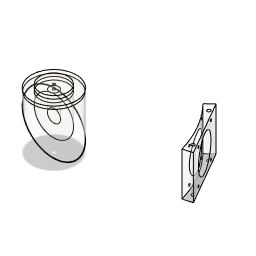
cage v11 (Autodesk Fusion 360 design; units mm, degrees)
Autodesk Fusion 360 part; units mm, degrees
note: some values were not read from the file. Chosen so that the rebuilt part matches the saved one: which bodies a step acts on; which face or edge a step refers to. Set by a fixed rule: which sketch regions a step uses.
(part 1 of 2)
sketch "Plate" plane through (0, 0, 0) normal (0, 1, 0) x (1, 0, 0) in component "Top Plate"
  circle A0 centre (0, 0) radius 228.6
  line L0 (0, 260.35) -> (0, 228.6) construction
  arc A1 (-273.05, -164.9615) -> (273.05, -164.9615) centre (0, 125.8796) ccw
  line L1 (-273.05, -164.9615) -> (-273.05, 0)
  line L2 (273.05, -164.9615) -> (273.05, 0)
  line L3 (0, 307.975) -> (126.2968, 242.0856)
  line L4 (0, 307.975) -> (-126.2968, 242.0856)
  circle A2 centre (0, 260.35) radius 3.302
  circle A3 centre (0, 0) radius 260.35 construction
  circle A4 centre (0, 260.35) radius 22.225 construction
  line L5 (0, -228.6) -> (0, -273.05) construction
  circle A5 centre (0, 0) radius 269.875 construction
  circle A6 centre (234.95, -132.7818) radius 22.225 construction
  circle A7 centre (234.95, -132.7818) radius 3.302
  circle A8 centre (-234.95, -132.7818) radius 3.302
  circle A9 centre (-234.95, -132.7818) radius 22.225 construction
  line L6 (-234.95, -132.7818) -> (234.95, -132.7818) construction
  arc A10 (-126.2968, 242.0856) -> (-273.05, 0) centre (0, 0) ccw
  arc A11 (273.05, 0) -> (126.2968, 242.0856) centre (0, 0) ccw
  line L7 (0, -228.6) -> (0, 0) construction
  line L8 (0, 0) -> (0, 228.6) construction
  line L9 (0, 260.35) -> (0, 307.975) construction
  line L10 (-126.2968, 242.0856) -> (126.2968, 242.0856) construction
  line L11 (-273.05, -164.9615) -> (0, 307.975) construction
  circle A12 centre (0, 0) radius 250.825 construction
  circle A13 centre (191.5577, 161.9223) radius 3.302
  circle A14 centre (236.0077, 84.9327) radius 3.302
  line L12 (191.5577, 161.9223) -> (236.0077, 84.9327) construction
  circle A15 centre (-236.0077, 84.9327) radius 3.302
  line L13 (-191.5577, 161.9223) -> (-236.0077, 84.9327) construction
  circle A16 centre (-191.5577, 161.9223) radius 3.302
  circle A17 centre (44.45, -246.855) radius 3.302
  line L14 (-44.45, -246.855) -> (44.45, -246.855) construction
  circle A18 centre (-44.45, -246.855) radius 3.302
  line L15 (213.7827, 123.4275) -> (0, -246.855) construction
  line L16 (0, -246.855) -> (-213.7827, 123.4275) construction
  line L17 (-213.7827, 123.4275) -> (213.7827, 123.4275) construction
  point P0 (0, -246.855)
  point P1 (-213.7827, 123.4275)
  point P2 (213.7827, 123.4275)
  dimension "d16_2" = 457.2
  dimension "d19_2" = 546.1
  dimension "d22_2" = 79.375
  dimension "d24_2" = 31.75
  dimension "d160_1" = 539.75
  dimension "d162_1" = 6.604
  dimension "d163_1" = 6.604
  dimension "d164_1" = 469.9
  dimension "d165_1" = 44.45
  dimension "d166_1" = 44.45
  dimension "d167_1" = 44.45
  dimension "d168_1" = 44.45
  dimension "d169_1" = 546.1
  dimension "d171_1" = 501.65
  dimension "d172_1" = 6.604
  dimension "d174_1" = 6.604
  dimension "d175_1" = 88.9
  dimension "d176_1" = 6.604
  dimension "d177_1" = 6.604
  dimension "d178_1" = 88.9
  dimension "d179_1" = 6.604
  dimension "d180_1" = 6.604
  dimension "d181_1" = 88.9
  dimension "d350" = 6.604
  constraint coincident A0.centre A3.centre
  constraint coincident A0 L0.end
  constraint vertical L0
  constraint concentric A0 A3
  constraint coincident L0.start A3
  constraint coincident A0 L5.start
  constraint midpoint A1 L5.end
  constraint vertical L5
  constraint coincident A5 A6.centre
  constraint concentric A6 A7
  constraint concentric A8 A9
  constraint coincident A8.centre A9.centre
  constraint coincident A6.centre A7.centre
  constraint horizontal L6
  constraint coincident A5 A8.centre
  constraint vertical L1
  constraint vertical L2
  constraint tangent L4 A10
  constraint tangent L3 A11
  constraint vertical L7
  constraint coincident L0.start A2.centre
  constraint vertical L9
  constraint collinear L0 L8
  constraint horizontal L10
  constraint tangent L1 A10
  constraint concentric A5 A12
  constraint coincident A12 A13.centre
  constraint coincident A12 A14.centre
  constraint coincident A13.centre L12.start
  constraint coincident A14.centre L12.end
  constraint coincident L13.start A16.centre
  constraint coincident A15.centre L13.end
  constraint coincident L14.start A18.centre
  constraint coincident A17.centre L14.end
  constraint coincident A12 A15.centre
  constraint coincident A12 L13.start
  constraint coincident A12 A17.centre
  constraint coincident A12 L14.start
  constraint midpoint L14 P0
  constraint coincident L5 P0
  constraint midpoint L13 P1
  constraint midpoint L12 P2
  constraint coincident P2 L15.start
  constraint coincident P0 L15.end
  constraint coincident P1 L16.end
  constraint equal L16 L17
  constraint equal L15 L16
  measures "d16_2" diameter of A0
  measures "d19_2" distance of A1.start A1.end
  measures "d22_2" distance of L3.start L0.end
  measures "d24_2" distance of L0.end L0.start
  measures "d160_1" diameter of A5
  measures "d162_1" diameter of A7
  measures "d163_1" diameter of A8
  measures "d164_1" distance of A8.centre A6.centre
  measures "d165_1" diameter of A9
  measures "d166_1" diameter of A6
  measures "d167_1" distance of L5.start L5.end
  measures "d168_1" diameter of A4
  measures "d169_1" distance of A1.start L3.start
  measures "d171_1" diameter of A12
  measures "d172_1" diameter of A13
  measures "d174_1" diameter of A14
  measures "d175_1" distance of A13.centre A14.centre
  measures "d176_1" diameter of A16
  measures "d177_1" diameter of A15
  measures "d178_1" distance of L13.start A15.centre
  measures "d179_1" diameter of A18
  measures "d180_1" diameter of A17
  measures "d181_1" distance of L14.start A17.centre
  measures "d350" diameter of A2
extrude "Extrude4" add sketch "Plate" along normal blind 19.05 makes body 1 in component "Top Plate"
sketch "Sketch1" plane through (0, 0, 0) normal (1, 0, 0) x (0, 0, -1) in component "Slice1"
  line L0 (-339.5498, 170.2069) -> (354.2377, 170.2069)
  line L1 (354.2377, 170.2069) -> (354.2377, -114.9113)
  line L2 (354.2377, -114.9113) -> (-339.5498, -114.9113)
  line L3 (-339.5498, -114.9113) -> (-339.5498, 170.2069)
  constraint horizontal L0
  constraint vertical L1
  constraint horizontal L2
  constraint vertical L3
extrude "Extrude1" add sketch "Sketch1" along normal blind 228.6 separate body makes body 2 in component "Slice1"
sketch "Sketch1 (2)" plane through (0, 0, 0) normal (1, 0, 0) x (0, 0, -1) in component "Slice2"
  line L0 (-339.5498, 170.2069) -> (354.2377, 170.2069)
  line L1 (354.2377, 170.2069) -> (354.2377, -114.9113)
  line L2 (354.2377, -114.9113) -> (-339.5498, -114.9113)
  line L3 (-339.5498, -114.9113) -> (-339.5498, 170.2069)
  constraint horizontal L0
  constraint vertical L1
  constraint horizontal L2
  constraint vertical L3
extrude "Extrude1'" add sketch "Sketch1 (2)" along normal blind 177.8 separate body makes body 3 in component "Slice2"
split "Split3" by plane through (0, 0, 0) normal (0.707107, 0, 0.707107) bodies 1 makes body 4 at (56.2654, 0, -258.2251) in component "Top Plate"
split "Split4" by plane through (0, 0, 0) normal (0.707107, 0, -0.707107) bodies 4 1 makes body 6 at (178.8171, 0, 204.0038) makes body 5 at (-261.2405, 0, 98.6008) in component "Top Plate"
copy_body "Body->Comp5" bodies 1 removing the originals makes body 7 in component "right (1)"
copy_body "Body->Comp6" bodies 4 removing the originals makes body 8 in component "front (1)"
copy_body "Body->Comp7" bodies 6 removing the originals makes body 9 in component "rear (1)"
copy_body "Body->Comp8" bodies 5 removing the originals makes body 10 in component "left (1)"
split "Split1" by plane through (0, 0, 0) normal (1, 0, 0) bodies 9 makes body 11 at (171.3232, 0, 210.5758) in component "rear (1)"
copy_body "Body->Comp1" bodies 9 removing the originals makes body 12 in component "left (2)"
copy_body "Body->Comp2" bodies 11 removing the originals makes body 13 in component "right (2)"
sketch "Sketch1 (3)" plane through (0, 0, 0) normal (1, 0, 0) x (0, 0, -1) in component "left (2)"
  line L0 (-273.05, 0) -> (-228.6, 0)
  line L1 (-228.6, 0) -> (-228.6, 19.05)
  line L2 (-228.6, 19.05) -> (-273.05, 19.05)
  line L3 (-273.05, 19.05) -> (-273.05, 0)
  line L4 (-266.7, 12.7) -> (-234.95, 12.7)
  line L5 (-234.95, 12.7) -> (-234.95, 6.35)
  line L6 (-234.95, 6.35) -> (-266.7, 6.35)
  line L7 (-266.7, 6.35) -> (-266.7, 12.7)
  line L8 (-256.54, 12.7) -> (-256.54, 19.05) construction
  line L9 (-241.3, 6.35) -> (-241.3, 0) construction
  line L10 (-234.95, 10.16) -> (-228.6, 10.16) construction
  line L11 (-266.7, 7.62) -> (-273.05, 7.62) construction
  dimension "d194" = 6.35
  dimension "d195" = 6.35
  dimension "d196" = 31.75
  dimension "d197" = 6.35
  constraint horizontal L4
  constraint vertical L5
  constraint horizontal L6
  constraint vertical L7
  constraint coincident L4 L8.start
  constraint coincident L2 L8.end
  constraint perpendicular L2 L8
  constraint coincident L6 L9.start
  constraint coincident L0 L9.end
  constraint perpendicular L0 L9
  constraint coincident L5 L10.start
  constraint coincident L1 L10.end
  constraint perpendicular L1 L10
  constraint coincident L7 L11.start
  constraint coincident L3 L11.end
  constraint perpendicular L3 L11
  constraint equal L10 L11
  constraint equal L8 L9
  measures "d194" distance of L8.start L8.end
  measures "d195" distance of L10.start L10.end
  measures "d196" distance of L5.end L6.end
  measures "d197" distance of L4.end L5.end
extrude "Extrude1''" cut sketch "Sketch1 (3)" against normal blind 12.7 contours L4 L5 L6 L7 bodies 12 in component "left (2)"
sketch "Sketch1 (4)" plane through (0, 0, 0) normal (-1, 0, 0) x (0, 0, 1) in component "right (2)"
  line L0 (228.6, 0) -> (273.05, 0)
  line L1 (273.05, 0) -> (273.05, 19.05)
  line L2 (273.05, 19.05) -> (228.6, 19.05)
  line L3 (228.6, 19.05) -> (228.6, 0)
  line L4 (234.95, 12.7) -> (266.7, 12.7)
  line L5 (266.7, 12.7) -> (266.7, 6.35)
  line L6 (266.7, 6.35) -> (234.95, 6.35)
  line L7 (234.95, 6.35) -> (234.95, 12.7)
  line L8 (240.9533, 6.35) -> (240.9533, 0) construction
  line L9 (256.54, 12.7) -> (256.54, 19.05) construction
  line L10 (266.7, 6.1597) -> (273.05, 6.1597) construction
  line L11 (234.95, 11.1721) -> (228.6, 11.1721) construction
  dimension "d200" = 6.35
  dimension "d201" = 6.35
  dimension "d202" = 31.75
  dimension "d203" = 6.35
  constraint horizontal L4
  constraint vertical L5
  constraint horizontal L6
  constraint vertical L7
  constraint coincident L6 L8.start
  constraint coincident L0 L8.end
  constraint perpendicular L0 L8
  constraint coincident L4 L9.start
  constraint coincident L2 L9.end
  constraint perpendicular L2 L9
  constraint coincident L5 L10.start
  constraint coincident L1 L10.end
  constraint perpendicular L1 L10
  constraint coincident L7 L11.start
  constraint coincident L3 L11.end
  constraint perpendicular L3 L11
  constraint equal L10 L11
  constraint equal L8 L9
  measures "d200" distance of L11.start L11.end
  measures "d201" distance of L8.start L8.end
  measures "d202" distance of L4.start L4.end
  measures "d203" distance of L4.start L6.end
extrude "Extrude1'''" cut sketch "Sketch1 (4)" against normal blind 12.7 contours L4 L5 L6 L7 bodies 13 in component "right (2)"
sketch "Sketch1 (5)" plane through (0, 6.35, 0) normal (0, 1, 0) x (-1, 0, 0) in component "Connector"
  line L0 (0, 266.7) -> (0, 234.95)
  line L1 (0, 234.95) -> (12.7, 234.95)
  line L2 (12.7, 234.95) -> (12.7, 266.7)
  line L3 (12.7, 266.7) -> (0, 266.7)
  line L4 (12.7, 266.192) -> (-12.192, 266.192)
  line L5 (-12.192, 266.192) -> (-12.192, 234.95)
  line L6 (-12.192, 234.95) -> (12.7, 234.95)
  line L7 (12.7, 234.95) -> (12.7, 266.192)
  dimension "d206" = 31.242
  dimension "d207" = 24.892
  constraint horizontal L4
  constraint vertical L5
  constraint horizontal L6
  constraint vertical L7
  constraint coincident L1.end L2.start
  measures "d206" distance of L1.end L4.start
  measures "d207" distance of L1.end L5.end
extrude "Extrude1''''" add sketch "Sketch1 (5)" along normal blind 5.715 separate body contours L0 L1 L2 L4 L6 L7 | L0 L4 L5 L6 makes body 14 in component "Connector"
sketch "Sketch2" plane through (0, 0, 0) normal (0.707107, 0, -0.707107) x (-0.707107, 0, -0.707107) in component "right (2)"
  line L0 (-228.6, 19.05) -> (-299.8624, 19.05)
  line L1 (-299.8624, 19.05) -> (-299.8624, 0)
  line L2 (-299.8624, 0) -> (-228.6, 0)
  line L3 (-228.6, 0) -> (-228.6, 19.05)
  line L4 (-293.5124, 12.7) -> (-234.95, 12.7)
  line L5 (-234.95, 12.7) -> (-234.95, 6.35)
  line L6 (-234.95, 6.35) -> (-293.5124, 6.35)
  line L7 (-293.5124, 6.35) -> (-293.5124, 12.7)
  line L8 (-276.86, 12.7) -> (-276.86, 19.05) construction
  line L9 (-293.5124, 9.3745) -> (-299.8624, 9.3745) construction
  line L10 (-248.92, 6.35) -> (-248.92, 0) construction
  line L11 (-234.95, 7.62) -> (-228.6, 7.62) construction
  dimension "d210" = 6.35
  dimension "d211" = 6.35
  constraint horizontal L4
  constraint vertical L5
  constraint horizontal L6
  constraint vertical L7
  constraint coincident L4 L8.start
  constraint coincident L0 L8.end
  constraint perpendicular L4 L8
  constraint coincident L7 L9.start
  constraint coincident L1 L9.end
  constraint perpendicular L1 L9
  constraint coincident L6 L10.start
  constraint coincident L2 L10.end
  constraint perpendicular L2 L10
  constraint coincident L5 L11.start
  constraint coincident L3 L11.end
  constraint perpendicular L3 L11
  constraint equal L9 L11
  constraint equal L8 L10
  measures "d210" distance of L8.start L8.end
  measures "d211" distance of L9.start L9.end
extrude "Extrude2" cut sketch "Sketch2" against normal blind 12.7 contours L4 L5 L6 L7 bodies 13 in component "right (2)"
sketch "Sketch3" plane through (0, 0, 0) normal (-0.707107, 0, -0.707107) x (-0.707107, 0, 0.707107) in component "left (2)"
  line L0 (299.8624, 0) -> (299.8624, 19.05)
  line L1 (299.8624, 19.05) -> (228.6, 19.05)
  line L2 (228.6, 19.05) -> (228.6, 0)
  line L3 (228.6, 0) -> (299.8624, 0)
  line L4 (234.95, 12.7) -> (293.5124, 12.7)
  line L5 (293.5124, 12.7) -> (293.5124, 6.35)
  line L6 (293.5124, 6.35) -> (234.95, 6.35)
  line L7 (234.95, 6.35) -> (234.95, 12.7)
  line L8 (248.92, 12.7) -> (248.92, 19.05) construction
  line L9 (284.48, 6.35) -> (284.48, 0) construction
  line L10 (293.5124, 10.16) -> (299.8624, 10.16) construction
  line L11 (234.95, 7.62) -> (228.6, 7.62) construction
  dimension "d214" = 6.35
  dimension "d215" = 6.35
  constraint horizontal L4
  constraint vertical L5
  constraint horizontal L6
  constraint vertical L7
  constraint coincident L4 L8.start
  constraint coincident L1 L8.end
  constraint perpendicular L1 L8
  constraint coincident L6 L9.start
  constraint coincident L3 L9.end
  constraint perpendicular L3 L9
  constraint coincident L5 L10.start
  constraint coincident L0 L10.end
  constraint perpendicular L0 L10
  constraint coincident L7 L11.start
  constraint coincident L2 L11.end
  constraint perpendicular L2 L11
  constraint equal L10 L11
  constraint equal L8 L9
  measures "d214" distance of L11.start L11.end
  measures "d215" distance of L9.start L9.end
extrude "Extrude2'" cut sketch "Sketch3" against normal blind 12.7 contours L4 L5 L6 L7 bodies 12 in component "left (2)"
sketch "Sketch1 (6)" plane through (0, 0, 0) normal (-0.707107, 0, 0.707107) x (0.707107, 0, 0.707107) in component "right (1)"
  line L0 (299.8624, 19.05) -> (228.6, 19.05)
  line L1 (228.6, 19.05) -> (228.6, 0)
  line L2 (228.6, 0) -> (299.8624, 0)
  line L3 (299.8624, 0) -> (299.8624, 19.05)
  line L4 (234.95, 12.7) -> (293.5124, 12.7)
  line L5 (293.5124, 12.7) -> (293.5124, 6.35)
  line L6 (293.5124, 6.35) -> (234.95, 6.35)
  line L7 (234.95, 6.35) -> (234.95, 12.7)
  line L8 (234.95, 8.89) -> (228.6, 8.89) construction
  line L9 (250.8852, 6.35) -> (250.8852, 0) construction
  line L10 (262.89, 12.7) -> (262.89, 19.05) construction
  line L11 (293.5124, 11.5709) -> (299.8624, 11.5709) construction
  dimension "d218" = 6.35
  dimension "d219" = 6.35
  dimension "d249" = 58.5624
  dimension "d250" = 6.35
  constraint horizontal L4
  constraint vertical L5
  constraint horizontal L6
  constraint vertical L7
  constraint coincident L7 L8.start
  constraint coincident L1 L8.end
  constraint perpendicular L1 L8
  constraint coincident L6 L9.start
  constraint coincident L2 L9.end
  constraint perpendicular L2 L9
  constraint coincident L4 L10.start
  constraint coincident L0 L10.end
  constraint perpendicular L0 L10
  constraint coincident L5 L11.start
  constraint coincident L3 L11.end
  constraint perpendicular L3 L11
  constraint equal L9 L10
  constraint equal L8 L11
  measures "d218" distance of L11.start L11.end
  measures "d219" distance of L10.start L10.end
  measures "d249" distance of L4.start L4.end
  measures "d250" distance of L4.start L6.end
extrude "Extrude1'''''" cut sketch "Sketch1 (6)" against normal blind 12.7 contours L4 L5 L6 L7 bodies 7 in component "right (1)"
sketch "Sketch2 (2)" plane through (0, 0, 0) normal (-0.707107, 0, -0.707107) x (-0.707107, 0, 0.707107) in component "right (1)"
  line L0 (-273.05, 19.05) -> (-273.05, 0)
  line L1 (-273.05, 0) -> (-228.6, 0)
  line L2 (-228.6, 0) -> (-228.6, 19.05)
  line L3 (-228.6, 19.05) -> (-273.05, 19.05)
  line L4 (-266.7, 12.7) -> (-234.95, 12.7)
  line L5 (-234.95, 12.7) -> (-234.95, 6.35)
  line L6 (-234.95, 6.35) -> (-266.7, 6.35)
  line L7 (-266.7, 6.35) -> (-266.7, 12.7)
  line L8 (-266.7, 7.62) -> (-273.05, 7.62) construction
  line L9 (-242.7847, 12.7) -> (-242.7847, 19.05) construction
  line L10 (-234.95, 12.7) -> (-228.6, 12.7) construction
  line L11 (-256.54, 6.35) -> (-256.54, 0) construction
  dimension "d222" = 6.35
  dimension "d223" = 6.35
  constraint horizontal L4
  constraint vertical L5
  constraint horizontal L6
  constraint vertical L7
  constraint coincident L7 L8.start
  constraint coincident L0 L8.end
  constraint perpendicular L0 L8
  constraint coincident L4 L9.start
  constraint coincident L3 L9.end
  constraint perpendicular L3 L9
  constraint coincident L5 L4.end
  constraint coincident L2 L10.end
  constraint perpendicular L2 L10
  constraint coincident L6 L11.start
  constraint coincident L1 L11.end
  constraint perpendicular L1 L11
  constraint equal L9 L11
  constraint equal L8 L10
  measures "d222" distance of L8.start L8.end
  measures "d223" distance of L11.start L11.end
extrude "Extrude2''" cut sketch "Sketch2 (2)" against normal blind 12.7 contours L4 L5 L6 L7 bodies 7 in component "right (1)"
sketch "Sketch1 (7)" plane through (0, 0, 0) normal (0.707107, 0, 0.707107) x (0.707107, 0, -0.707107) in component "left (1)"
  line L0 (-299.8624, 19.05) -> (-299.8624, 0)
  line L1 (-299.8624, 0) -> (-228.6, 0)
  line L2 (-228.6, 0) -> (-228.6, 19.05)
  line L3 (-228.6, 19.05) -> (-299.8624, 19.05)
  line L4 (-293.5124, 12.7) -> (-234.95, 12.7)
  line L5 (-234.95, 12.7) -> (-234.95, 6.35)
  line L6 (-234.95, 6.35) -> (-293.5124, 6.35)
  line L7 (-293.5124, 6.35) -> (-293.5124, 12.7)
  line L8 (-234.95, 8.376) -> (-228.6, 8.376) construction
  line L9 (-293.5124, 9.5249) -> (-299.8624, 9.5249) construction
  line L10 (-284.8839, 19.05) -> (-284.8839, 12.7) construction
  line L11 (-271.78, 6.35) -> (-271.78, 0) construction
  dimension "d226" = 6.35
  dimension "d227" = 6.35
  dimension "d247" = 58.5624
  dimension "d248" = 6.35
  constraint horizontal L4
  constraint vertical L5
  constraint horizontal L6
  constraint vertical L7
  constraint coincident L5 L8.start
  constraint perpendicular L5 L8
  constraint coincident L7 L9.start
  constraint coincident L0 L9.end
  constraint perpendicular L0 L9
  constraint coincident L3 L10.start
  constraint coincident L4 L10.end
  constraint perpendicular L4 L10
  constraint coincident L6 L11.start
  constraint coincident L1 L11.end
  constraint perpendicular L1 L11
  constraint equal L10 L11
  constraint equal L8 L9
  constraint coincident L2 L8.end
  measures "d226" distance of L9.start L9.end
  measures "d227" distance of L10.start L10.end
  measures "d247" distance of L4.start L4.end
  measures "d248" distance of L4.start L6.end
extrude "Extrude1''''''" cut sketch "Sketch1 (7)" against normal blind 12.7 contours L4 L5 L6 L7 bodies 10 in component "left (1)"
sketch "Sketch2 (3)" plane through (0, 0, 0) normal (0.707107, 0, -0.707107) x (-0.707107, 0, -0.707107) in component "left (1)"
  line L0 (273.05, 19.05) -> (228.6, 19.05)
  line L1 (228.6, 19.05) -> (228.6, 0)
  line L2 (228.6, 0) -> (273.05, 0)
  line L3 (273.05, 0) -> (273.05, 19.05)
  line L4 (234.95, 12.7) -> (266.7, 12.7)
  line L5 (266.7, 12.7) -> (266.7, 6.35)
  line L6 (266.7, 6.35) -> (234.95, 6.35)
  line L7 (234.95, 6.35) -> (234.95, 12.7)
  line L8 (243.84, 12.7) -> (243.84, 19.05) construction
  line L9 (261.9443, 6.35) -> (261.9443, 0) construction
  line L10 (266.7, 9.6711) -> (273.05, 9.6711) construction
  line L11 (234.95, 7.62) -> (228.6, 7.62) construction
  dimension "d230" = 6.35
  dimension "d231" = 6.35
  constraint horizontal L4
  constraint vertical L5
  constraint horizontal L6
  constraint vertical L7
  constraint coincident L4 L8.start
  constraint coincident L0 L8.end
  constraint perpendicular L0 L8
  constraint coincident L6 L9.start
  constraint perpendicular L6 L9
  constraint coincident L5 L10.start
  constraint coincident L3 L10.end
  constraint perpendicular L3 L10
  constraint coincident L7 L11.start
  constraint coincident L1 L11.end
  constraint perpendicular L1 L11
  constraint equal L10 L11
  constraint equal L8 L9
  constraint coincident L2 L9.end
  measures "d230" distance of L11.start L11.end
  measures "d231" distance of L8.start L8.end
extrude "Extrude2'''" cut sketch "Sketch2 (3)" against normal blind 12.7 contours L4 L5 L6 L7 bodies 10 in component "left (1)"
sketch "Sketch1 (8)" plane through (0, 0, 0) normal (0.707107, 0, 0.707107) x (0.707107, 0, -0.707107) in component "front (1)"
  line L0 (273.05, 0) -> (273.05, 19.05)
  line L1 (273.05, 19.05) -> (228.6, 19.05)
  line L2 (228.6, 19.05) -> (228.6, 0)
  line L3 (228.6, 0) -> (273.05, 0)
  line L4 (234.95, 12.7) -> (266.7, 12.7)
  line L5 (266.7, 12.7) -> (266.7, 6.35)
  line L6 (266.7, 6.35) -> (234.95, 6.35)
  line L7 (234.95, 6.35) -> (234.95, 12.7)
  line L8 (234.95, 11.43) -> (228.6, 11.43) construction
  line L9 (241.3, 12.7) -> (241.3, 19.05) construction
  line L10 (245.7528, 6.35) -> (245.7528, 0) construction
  line L11 (266.7, 9.525) -> (273.05, 9.525) construction
  dimension "d234" = 6.35
  dimension "d235" = 6.35
  dimension "d242" = 6.35
  dimension "d243" = 31.75
  constraint horizontal L4
  constraint vertical L5
  constraint horizontal L6
  constraint vertical L7
  constraint coincident L7 L8.start
  constraint coincident L2 L8.end
  constraint perpendicular L2 L8
  constraint coincident L4 L9.start
  constraint coincident L1 L9.end
  constraint perpendicular L1 L9
  constraint coincident L6 L10.start
  constraint coincident L3 L10.end
  constraint perpendicular L3 L10
  constraint coincident L5 L11.start
  constraint perpendicular L5 L11
  constraint equal L9 L10
  constraint equal L8 L11
  constraint midpoint L0 L11.end
  measures "d234" distance of L11.start L11.end
  measures "d235" distance of L10.start L10.end
  measures "d242" distance of L4.start L6.end
  measures "d243" distance of L4.start L4.end
extrude "Extrude1'''''''" cut sketch "Sketch1 (8)" against normal blind 12.7 contours L4 L5 L6 L7 bodies 8 in component "front (1)"
sketch "Sketch2 (4)" plane through (0, 0, 0) normal (-0.707107, 0, 0.707107) x (0.707107, 0, 0.707107) in component "front (1)"
  line L0 (-228.6, 19.05) -> (-273.05, 19.05)
  line L1 (-273.05, 19.05) -> (-273.05, 0)
  line L2 (-273.05, 0) -> (-228.6, 0)
  line L3 (-228.6, 0) -> (-228.6, 19.05)
  line L4 (-266.7, 12.7) -> (-234.95, 12.7)
  line L5 (-234.95, 12.7) -> (-234.95, 6.35)
  line L6 (-234.95, 6.35) -> (-266.7, 6.35)
  line L7 (-266.7, 6.35) -> (-266.7, 12.7)
  line L8 (-241.3, 12.7) -> (-241.3, 19.05) construction
  line L9 (-234.95, 10.16) -> (-228.6, 10.16) construction
  line L10 (-266.7, 9.525) -> (-273.05, 9.525) construction
  line L11 (-256.54, 6.35) -> (-256.54, 0) construction
  dimension "d238" = 6.35
  dimension "d239" = 6.35
  dimension "d244" = 6.35
  dimension "d245" = 31.75
  constraint horizontal L4
  constraint vertical L5
  constraint horizontal L6
  constraint vertical L7
  constraint coincident L4 L8.start
  constraint coincident L0 L8.end
  constraint perpendicular L0 L8
  constraint coincident L5 L9.start
  constraint coincident L3 L9.end
  constraint perpendicular L3 L9
  constraint midpoint L7 L10.start
  constraint coincident L1 L10.end
  constraint perpendicular L1 L10
  constraint coincident L6 L11.start
  constraint coincident L2 L11.end
  constraint perpendicular L2 L11
  constraint equal L8 L11
  constraint equal L9 L10
  measures "d238" distance of L10.start L10.end
  measures "d239" distance of L11.start L11.end
  measures "d244" distance of L4.end L5.end
  measures "d245" distance of L5.end L6.end
extrude "Extrude2''''" cut sketch "Sketch2 (4)" against normal blind 12.7 contours L4 L5 L6 L7 bodies 8 in component "front (1)"
sketch "Sketch1 (9)" plane through (0, 6.35, 0) normal (0, 1, 0) x (-1, 0, 0) in component "LargeConnector"
  line L0 (-207.5446, 207.5446) -> (-166.1347, 166.1347)
  line L1 (-166.1347, 166.1347) -> (-157.1545, 175.115)
  line L2 (-157.1545, 175.115) -> (-198.5644, 216.5249)
  line L3 (-198.5644, 216.5249) -> (-207.5446, 207.5446)
  line L4 (-219.9225, 194.7967) -> (-178.7929, 153.6671)
  line L5 (-178.7929, 153.6671) -> (-196.3942, 136.0658)
  line L6 (-196.3942, 136.0658) -> (-237.5238, 177.1954)
  line L7 (-237.5238, 177.1954) -> (-219.9225, 194.7967)
  dimension "d267" = 12.7
  dimension "d268" = 12.7
  dimension "d269" = 58.5624
  dimension "d270" = 58.166
  dimension "d271" = 24.892
  constraint parallel L1 L5
  constraint parallel L3 L7
  constraint parallel L0 L6
  constraint parallel L2 L4
  measures "d267" distance of L0.start L2.end
  measures "d268" distance of L0.end L1.end
  measures "d269" distance of L1.end L2.end
  measures "d270" distance of L4.start L4.end
  measures "d271" distance of L4.end L5.end
extrude "Extrude1''''''''" add sketch "Sketch1 (9)" along normal blind 5.842 separate body contours L4 L5 L6 L7 makes body 15 in component "LargeConnector"
fillet "Fillet1" radius 1.27 1 edges at (237.5238, 9.271, 177.1954) on bodies 15 in component "LargeConnector"
fillet "Fillet2" radius 1.27 3 edges at (228.2741, 12.192, 186.4451) (236.9977, 12.192, 177.1954) (216.51, 12.192, 156.1816) on bodies 15 in component "LargeConnector"
fillet "Fillet3" radius 1.27 3 edges at (216.51, 6.35, 156.1816) (236.9977, 6.35, 177.1954) (228.2741, 6.35, 186.4451) on bodies 15 in component "LargeConnector"
fillet "Fillet4" radius 1.27 5 edges at (198.9087, 12.192, 173.7829) (219.6595, 11.82, 194.5337) (219.9225, 9.271, 194.7967) (219.6595, 6.722, 194.5337) (198.9087, 6.35, 173.7829) on bodies 15 in component "LargeConnector"
fillet "Fillet5" radius 1.27 8 edges at (196.3942, 9.271, 136.0658) (196.1312, 11.82, 136.3289) (187.5936, 12.192, 144.8665) (179.0559, 11.82, 153.4041) (178.7929, 9.271, 153.6671) (179.0559, 6.722, 153.4041) (187.5936, 6.35, 144.8665) (196.1312, 6.722, 136.3289) on bodies 15 in component "LargeConnector"
fillet "Fillet1'" radius 1.27 1 edges at (-12.7, 9.2075, 266.192) on bodies 14 in component "Connector"
fillet "Fillet2'" radius 1.27 1 edges at (-12.7, 9.2075, 234.95) on bodies 14 in component "Connector"
fillet "Fillet3'" radius 1.27 5 edges at (0.381, 12.065, 234.95) (-12.328, 12.065, 235.322) (-12.7, 12.065, 250.571) (-12.328, 12.065, 265.82) (0.381, 12.065, 266.192) on bodies 14 in component "Connector"
fillet "Fillet4'" radius 1.27 5 edges at (12.192, 8.5725, 266.192) (12.192, 11.693, 265.82) (12.192, 12.065, 250.571) (12.192, 11.693, 235.322) (12.192, 8.5725, 234.95) on bodies 14 in component "Connector"
fillet "Fillet5'" radius 1.27 8 edges at (-0.254, 6.35, 266.192) (11.82, 6.35, 265.82) (12.192, 6.35, 250.571) (11.82, 6.35, 235.322) (-0.254, 6.35, 234.95) (-12.328, 6.35, 235.322) (-12.7, 6.35, 250.571) (-12.328, 6.35, 265.82) on bodies 14 in component "Connector"
sketch "Plate (2)" plane through (0, 0, 0) normal (0, 1, 0) x (1, 0, 0) in component "Bottom Plate"
  circle A0 centre (0, 0) radius 228.6
  line L0 (0, 260.35) -> (0, 228.6) construction
  arc A1 (-273.05, -164.9615) -> (273.05, -164.9615) centre (0, 125.8796) ccw
  line L1 (-273.05, -164.9615) -> (-273.05, 0)
  line L2 (273.05, -164.9615) -> (273.05, 0)
  line L3 (0, 307.975) -> (126.2968, 242.0856)
  line L4 (0, 307.975) -> (-126.2968, 242.0856)
  circle A2 centre (0, 260.35) radius 3.302
  circle A3 centre (0, 0) radius 260.35 construction
  circle A4 centre (0, 260.35) radius 22.225 construction
  line L5 (0, -228.6) -> (0, -273.05) construction
  circle A5 centre (0, 0) radius 269.875 construction
  circle A6 centre (234.95, -132.7818) radius 22.225 construction
  circle A7 centre (234.95, -132.7818) radius 3.302
  circle A8 centre (-234.95, -132.7818) radius 3.302
  circle A9 centre (-234.95, -132.7818) radius 22.225 construction
  line L6 (-234.95, -132.7818) -> (234.95, -132.7818) construction
  arc A10 (-126.2968, 242.0856) -> (-273.05, 0) centre (0, 0) ccw
  arc A11 (273.05, 0) -> (126.2968, 242.0856) centre (0, 0) ccw
  line L7 (0, -228.6) -> (0, 0) construction
  line L8 (0, 0) -> (0, 228.6) construction
  line L9 (0, 260.35) -> (0, 307.975) construction
  line L10 (-126.2968, 242.0856) -> (126.2968, 242.0856) construction
  line L11 (-273.05, -164.9615) -> (0, 307.975) construction
  circle A12 centre (0, 0) radius 250.825 construction
  circle A13 centre (191.5577, 161.9223) radius 3.302
  circle A14 centre (236.0077, 84.9327) radius 3.302
  line L12 (191.5577, 161.9223) -> (236.0077, 84.9327) construction
  circle A15 centre (-236.0077, 84.9327) radius 3.302
  line L13 (-191.5577, 161.9223) -> (-236.0077, 84.9327) construction
  circle A16 centre (-191.5577, 161.9223) radius 3.302
  circle A17 centre (44.45, -246.855) radius 3.302
  line L14 (-44.45, -246.855) -> (44.45, -246.855) construction
  circle A18 centre (-44.45, -246.855) radius 3.302
  line L15 (213.7827, 123.4275) -> (0, -246.855) construction
  line L16 (0, -246.855) -> (-213.7827, 123.4275) construction
  line L17 (-213.7827, 123.4275) -> (213.7827, 123.4275) construction
  circle A19 centre (-235.7042, -110.5696) radius 12.7
  circle A20 centre (235.7042, -110.5696) radius 12.7
  point P0 (0, -246.855)
  point P1 (-213.7827, 123.4275)
  point P2 (213.7827, 123.4275)
  dimension "d16_2_1" = 457.2
  dimension "d19_2_1" = 546.1
  dimension "d22_2_1" = 79.375
  dimension "d24_2_1" = 31.75
  dimension "d160_1_1" = 539.75
  dimension "d162_1_1" = 6.604
  dimension "d163_1_1" = 6.604
  dimension "d164_1_1" = 469.9
  dimension "d165_1_1" = 44.45
  dimension "d166_1_1" = 44.45
  dimension "d167_1_1" = 44.45
  dimension "d168_1_1" = 44.45
  dimension "d169_1_1" = 546.1
  dimension "d171_1_1" = 501.65
  dimension "d172_1_1" = 6.604
  dimension "d174_1_1" = 6.604
  dimension "d175_1_1" = 88.9
  dimension "d176_1_1" = 6.604
  dimension "d177_1_1" = 6.604
  dimension "d178_1_1" = 88.9
  dimension "d179_1_1" = 6.604
  dimension "d180_1_1" = 6.604
  dimension "d181_1_1" = 88.9
  dimension "d340" = 25.4
  dimension "d341" = 25.4
  dimension "d349" = 6.604
  constraint coincident A0.centre A3.centre
  constraint coincident A0 L0.end
  constraint vertical L0
  constraint concentric A0 A3
  constraint coincident L0.start A3
  constraint coincident A0 L5.start
  constraint midpoint A1 L5.end
  constraint vertical L5
  constraint coincident A5 A6.centre
  constraint concentric A6 A7
  constraint concentric A8 A9
  constraint coincident A8.centre A9.centre
  constraint coincident A6.centre A7.centre
  constraint horizontal L6
  constraint coincident A5 A8.centre
  constraint vertical L1
  constraint vertical L2
  constraint tangent L4 A10
  constraint tangent L3 A11
  constraint vertical L7
  constraint coincident L0.start A2.centre
  constraint vertical L9
  constraint collinear L0 L8
  constraint horizontal L10
  constraint tangent L1 A10
  constraint concentric A5 A12
  constraint coincident A12 A13.centre
  constraint coincident A12 A14.centre
  constraint coincident A13.centre L12.start
  constraint coincident A14.centre L12.end
  constraint coincident L13.start A16.centre
  constraint coincident A15.centre L13.end
  constraint coincident L14.start A18.centre
  constraint coincident A17.centre L14.end
  constraint coincident A12 A15.centre
  constraint coincident A12 L13.start
  constraint coincident A12 A17.centre
  constraint coincident A12 L14.start
  constraint midpoint L14 P0
  constraint coincident L5 P0
  constraint midpoint L13 P1
  constraint midpoint L12 P2
  constraint coincident P2 L15.start
  constraint coincident P0 L15.end
  constraint coincident P1 L16.end
  constraint equal L16 L17
  constraint equal L15 L16
  constraint coincident A9 A19.centre
  constraint coincident A3 A19.centre
  constraint coincident A6 A20.centre
  constraint coincident A3 A20.centre
  measures "d16_2_1" diameter of A0
  measures "d19_2_1" distance of A1.start A1.end
  measures "d22_2_1" distance of L3.start L0.end
  measures "d24_2_1" distance of L0.end L0.start
  measures "d160_1_1" diameter of A5
  measures "d162_1_1" diameter of A7
  measures "d163_1_1" diameter of A8
  measures "d164_1_1" distance of A8.centre A6.centre
  measures "d165_1_1" diameter of A9
  measures "d166_1_1" diameter of A6
  measures "d167_1_1" distance of L5.start L5.end
  measures "d168_1_1" diameter of A4
  measures "d169_1_1" distance of A1.start L3.start
  measures "d171_1_1" diameter of A12
  measures "d172_1_1" diameter of A13
  measures "d174_1_1" diameter of A14
  measures "d175_1_1" distance of A13.centre A14.centre
  measures "d176_1_1" diameter of A16
  measures "d177_1_1" diameter of A15
  measures "d178_1_1" distance of L13.start A15.centre
  measures "d179_1_1" diameter of A18
  measures "d180_1_1" diameter of A17
  measures "d181_1_1" distance of L14.start A17.centre
  measures "d340" diameter of A19
  measures "d341" diameter of A20
  measures "d349" diameter of A2
extrude "Extrude4'" add sketch "Plate (2)" along normal blind 19.05 separate body makes body 16 in component "Bottom Plate"
split "Split3'" by plane through (0, 0, 0) normal (0.707107, 0, 0.707107) bodies 16 makes body 17 at (56.2654, 0, -258.2251) in component "Bottom Plate"
split "Split4'" by plane through (0, 0, 0) normal (0.707107, 0, -0.707107) bodies 17 16 makes body 18 at (178.8171, 0, 204.0038) makes body 19 at (-216.5187, 0, 156.7439) in component "Bottom Plate"
copy_body "Body->Comp5'" bodies 16 removing the originals makes body 20 in component "right (1) (1)"
copy_body "Body->Comp6'" bodies 17 removing the originals makes body 21 in component "front (1) (1)"
copy_body "Body->Comp7'" bodies 18 removing the originals makes body 22 in component "rear (1) (1)"
copy_body "Body->Comp8'" bodies 19 removing the originals makes body 23 in component "left (1) (1)"
split "Split1'" by plane through (0, 0, 0) normal (1, 0, 0) bodies 22 makes body 24 at (171.3232, 0, 210.5758) in component "rear (1) (1)"
copy_body "Body->Comp1'" bodies 22 removing the originals makes body 25 in component "left (2) (1)"
copy_body "Body->Comp2'" bodies 24 removing the originals makes body 26 in component "right (2) (1)"
sketch "Sketch1 (10)" plane through (0, 0, 0) normal (1, 0, 0) x (0, 0, -1) in component "left (2) (1)"
  line L0 (-273.05, 0) -> (-228.6, 0)
  line L1 (-228.6, 0) -> (-228.6, 19.05)
  line L2 (-228.6, 19.05) -> (-273.05, 19.05)
  line L3 (-273.05, 19.05) -> (-273.05, 0)
  line L4 (-266.7, 12.7) -> (-234.95, 12.7)
  line L5 (-234.95, 12.7) -> (-234.95, 6.35)
  line L6 (-234.95, 6.35) -> (-266.7, 6.35)
  line L7 (-266.7, 6.35) -> (-266.7, 12.7)
  line L8 (-256.54, 12.7) -> (-256.54, 19.05) construction
  line L9 (-241.3, 6.35) -> (-241.3, 0) construction
  line L10 (-234.95, 10.16) -> (-228.6, 10.16) construction
  line L11 (-266.7, 7.62) -> (-273.05, 7.62) construction
  dimension "d194_1" = 6.35
  dimension "d195_1" = 6.35
  dimension "d196_1" = 31.75
  dimension "d197_1" = 6.35
  constraint horizontal L4
  constraint vertical L5
  constraint horizontal L6
  constraint vertical L7
  constraint coincident L4 L8.start
  constraint coincident L2 L8.end
  constraint perpendicular L2 L8
  constraint coincident L6 L9.start
  constraint coincident L0 L9.end
  constraint perpendicular L0 L9
  constraint coincident L5 L10.start
  constraint coincident L1 L10.end
  constraint perpendicular L1 L10
  constraint coincident L7 L11.start
  constraint coincident L3 L11.end
  constraint perpendicular L3 L11
  constraint equal L10 L11
  constraint equal L8 L9
  measures "d194_1" distance of L8.start L8.end
  measures "d195_1" distance of L10.start L10.end
  measures "d196_1" distance of L5.end L6.end
  measures "d197_1" distance of L4.end L5.end
extrude "Extrude1'''''''''" cut sketch "Sketch1 (10)" against normal blind 12.7 contours L4 L5 L6 L7 bodies 25 in component "left (2) (1)"
sketch "Sketch1 (11)" plane through (0, 0, 0) normal (-1, 0, 0) x (0, 0, 1) in component "right (2) (1)"
  line L0 (228.6, 0) -> (273.05, 0)
  line L1 (273.05, 0) -> (273.05, 19.05)
  line L2 (273.05, 19.05) -> (228.6, 19.05)
  line L3 (228.6, 19.05) -> (228.6, 0)
  line L4 (234.95, 12.7) -> (266.7, 12.7)
  line L5 (266.7, 12.7) -> (266.7, 6.35)
  line L6 (266.7, 6.35) -> (234.95, 6.35)
  line L7 (234.95, 6.35) -> (234.95, 12.7)
  line L8 (240.9533, 6.35) -> (240.9533, 0) construction
  line L9 (256.54, 12.7) -> (256.54, 19.05) construction
  line L10 (266.7, 6.1597) -> (273.05, 6.1597) construction
  line L11 (234.95, 11.1721) -> (228.6, 11.1721) construction
  dimension "d200_1" = 6.35
  dimension "d201_1" = 6.35
  dimension "d202_1" = 31.75
  dimension "d203_1" = 6.35
  constraint horizontal L4
  constraint vertical L5
  constraint horizontal L6
  constraint vertical L7
  constraint coincident L6 L8.start
  constraint coincident L0 L8.end
  constraint perpendicular L0 L8
  constraint coincident L4 L9.start
  constraint coincident L2 L9.end
  constraint perpendicular L2 L9
  constraint coincident L5 L10.start
  constraint coincident L1 L10.end
  constraint perpendicular L1 L10
  constraint coincident L7 L11.start
  constraint coincident L3 L11.end
  constraint perpendicular L3 L11
  constraint equal L10 L11
  constraint equal L8 L9
  measures "d200_1" distance of L11.start L11.end
  measures "d201_1" distance of L8.start L8.end
  measures "d202_1" distance of L4.start L4.end
  measures "d203_1" distance of L4.start L6.end
extrude "Extrude1''''''''''" cut sketch "Sketch1 (11)" against normal blind 12.7 contours L4 L5 L6 L7 bodies 26 in component "right (2) (1)"
sketch "Sketch1 (12)" plane through (0, 6.35, 0) normal (0, 1, 0) x (-1, 0, 0) in component "Connector (1)"
  line L0 (0, 266.7) -> (0, 234.95)
  line L1 (0, 234.95) -> (12.7, 234.95)
  line L2 (12.7, 234.95) -> (12.7, 266.7)
  line L3 (12.7, 266.7) -> (0, 266.7)
  line L4 (12.7, 266.192) -> (-12.192, 266.192)
  line L5 (-12.192, 266.192) -> (-12.192, 234.95)
  line L6 (-12.192, 234.95) -> (12.7, 234.95)
  line L7 (12.7, 234.95) -> (12.7, 266.192)
  dimension "d206_1" = 31.242
  dimension "d207_1" = 24.892
  constraint horizontal L4
  constraint vertical L5
  constraint horizontal L6
  constraint vertical L7
  constraint coincident L1.end L2.start
  measures "d206_1" distance of L1.end L4.start
  measures "d207_1" distance of L1.end L5.end
extrude "Extrude1'''''''''''" add sketch "Sketch1 (12)" along normal blind 5.715 separate body contours L0 L1 L2 L4 L6 L7 | L0 L4 L5 L6 makes body 27 in component "Connector (1)"
sketch "Sketch2 (5)" plane through (0, 0, 0) normal (0.707107, 0, -0.707107) x (-0.707107, 0, -0.707107) in component "right (2) (1)"
  line L0 (-228.6, 19.05) -> (-299.8624, 19.05)
  line L1 (-299.8624, 19.05) -> (-299.8624, 0)
  line L2 (-299.8624, 0) -> (-228.6, 0)
  line L3 (-228.6, 0) -> (-228.6, 19.05)
  line L4 (-293.5124, 12.7) -> (-234.95, 12.7)
  line L5 (-234.95, 12.7) -> (-234.95, 6.35)
  line L6 (-234.95, 6.35) -> (-293.5124, 6.35)
  line L7 (-293.5124, 6.35) -> (-293.5124, 12.7)
  line L8 (-276.86, 12.7) -> (-276.86, 19.05) construction
  line L9 (-293.5124, 9.3745) -> (-299.8624, 9.3745) construction
  line L10 (-248.92, 6.35) -> (-248.92, 0) construction
  line L11 (-234.95, 7.62) -> (-228.6, 7.62) construction
  dimension "d210_1" = 6.35
  dimension "d211_1" = 6.35
  constraint horizontal L4
  constraint vertical L5
  constraint horizontal L6
  constraint vertical L7
  constraint coincident L4 L8.start
  constraint coincident L0 L8.end
  constraint perpendicular L4 L8
  constraint coincident L7 L9.start
  constraint coincident L1 L9.end
  constraint perpendicular L1 L9
  constraint coincident L6 L10.start
  constraint coincident L2 L10.end
  constraint perpendicular L2 L10
  constraint coincident L5 L11.start
  constraint coincident L3 L11.end
  constraint perpendicular L3 L11
  constraint equal L9 L11
  constraint equal L8 L10
  measures "d210_1" distance of L8.start L8.end
  measures "d211_1" distance of L9.start L9.end
extrude "Extrude2'''''" cut sketch "Sketch2 (5)" against normal blind 12.7 contours L4 L5 L6 L7 bodies 26 in component "right (2) (1)"
sketch "Sketch3 (2)" plane through (0, 0, 0) normal (-0.707107, 0, -0.707107) x (-0.707107, 0, 0.707107) in component "left (2) (1)"
  line L0 (299.8624, 0) -> (299.8624, 19.05)
  line L1 (299.8624, 19.05) -> (228.6, 19.05)
  line L2 (228.6, 19.05) -> (228.6, 0)
  line L3 (228.6, 0) -> (299.8624, 0)
  line L4 (234.95, 12.7) -> (293.5124, 12.7)
  line L5 (293.5124, 12.7) -> (293.5124, 6.35)
  line L6 (293.5124, 6.35) -> (234.95, 6.35)
  line L7 (234.95, 6.35) -> (234.95, 12.7)
  line L8 (248.92, 12.7) -> (248.92, 19.05) construction
  line L9 (284.48, 6.35) -> (284.48, 0) construction
  line L10 (293.5124, 10.16) -> (299.8624, 10.16) construction
  line L11 (234.95, 7.62) -> (228.6, 7.62) construction
  dimension "d214_1" = 6.35
  dimension "d215_1" = 6.35
  constraint horizontal L4
  constraint vertical L5
  constraint horizontal L6
  constraint vertical L7
  constraint coincident L4 L8.start
  constraint coincident L1 L8.end
  constraint perpendicular L1 L8
  constraint coincident L6 L9.start
  constraint coincident L3 L9.end
  constraint perpendicular L3 L9
  constraint coincident L5 L10.start
  constraint coincident L0 L10.end
  constraint perpendicular L0 L10
  constraint coincident L7 L11.start
  constraint coincident L2 L11.end
  constraint perpendicular L2 L11
  constraint equal L10 L11
  constraint equal L8 L9
  measures "d214_1" distance of L11.start L11.end
  measures "d215_1" distance of L9.start L9.end
extrude "Extrude2''''''" cut sketch "Sketch3 (2)" against normal blind 12.7 contours L4 L5 L6 L7 bodies 25 in component "left (2) (1)"
sketch "Sketch1 (13)" plane through (0, 0, 0) normal (-0.707107, 0, 0.707107) x (0.707107, 0, 0.707107) in component "right (1) (1)"
  line L0 (299.8624, 19.05) -> (228.6, 19.05)
  line L1 (228.6, 19.05) -> (228.6, 0)
  line L2 (228.6, 0) -> (299.8624, 0)
  line L3 (299.8624, 0) -> (299.8624, 19.05)
  line L4 (234.95, 12.7) -> (293.5124, 12.7)
  line L5 (293.5124, 12.7) -> (293.5124, 6.35)
  line L6 (293.5124, 6.35) -> (234.95, 6.35)
  line L7 (234.95, 6.35) -> (234.95, 12.7)
  line L8 (234.95, 8.89) -> (228.6, 8.89) construction
  line L9 (250.8852, 6.35) -> (250.8852, 0) construction
  line L10 (262.89, 12.7) -> (262.89, 19.05) construction
  line L11 (293.5124, 11.5709) -> (299.8624, 11.5709) construction
  dimension "d218_1" = 6.35
  dimension "d219_1" = 6.35
  dimension "d249_1" = 58.5624
  dimension "d250_1" = 6.35
  constraint horizontal L4
  constraint vertical L5
  constraint horizontal L6
  constraint vertical L7
  constraint coincident L7 L8.start
  constraint coincident L1 L8.end
  constraint perpendicular L1 L8
  constraint coincident L6 L9.start
  constraint coincident L2 L9.end
  constraint perpendicular L2 L9
  constraint coincident L4 L10.start
  constraint coincident L0 L10.end
  constraint perpendicular L0 L10
  constraint coincident L5 L11.start
  constraint coincident L3 L11.end
  constraint perpendicular L3 L11
  constraint equal L9 L10
  constraint equal L8 L11
  measures "d218_1" distance of L11.start L11.end
  measures "d219_1" distance of L10.start L10.end
  measures "d249_1" distance of L4.start L4.end
  measures "d250_1" distance of L4.start L6.end
extrude "Extrude1''''''''''''" cut sketch "Sketch1 (13)" against normal blind 12.7 contours L4 L5 L6 L7 bodies 20 in component "right (1) (1)"
sketch "Sketch2 (6)" plane through (0, 0, 0) normal (-0.707107, 0, -0.707107) x (-0.707107, 0, 0.707107) in component "right (1) (1)"
  line L0 (-273.05, 19.05) -> (-273.05, 0)
  line L1 (-273.05, 0) -> (-228.6, 0)
  line L2 (-228.6, 0) -> (-228.6, 19.05)
  line L3 (-228.6, 19.05) -> (-273.05, 19.05)
  line L4 (-266.7, 12.7) -> (-234.95, 12.7)
  line L5 (-234.95, 12.7) -> (-234.95, 6.35)
  line L6 (-234.95, 6.35) -> (-266.7, 6.35)
  line L7 (-266.7, 6.35) -> (-266.7, 12.7)
  line L8 (-266.7, 7.62) -> (-273.05, 7.62) construction
  line L9 (-242.7847, 12.7) -> (-242.7847, 19.05) construction
  line L10 (-234.95, 12.7) -> (-228.6, 12.7) construction
  line L11 (-256.54, 6.35) -> (-256.54, 0) construction
  dimension "d222_1" = 6.35
  dimension "d223_1" = 6.35
  constraint horizontal L4
  constraint vertical L5
  constraint horizontal L6
  constraint vertical L7
  constraint coincident L7 L8.start
  constraint coincident L0 L8.end
  constraint perpendicular L0 L8
  constraint coincident L4 L9.start
  constraint coincident L3 L9.end
  constraint perpendicular L3 L9
  constraint coincident L5 L4.end
  constraint coincident L2 L10.end
  constraint perpendicular L2 L10
  constraint coincident L6 L11.start
  constraint coincident L1 L11.end
  constraint perpendicular L1 L11
  constraint equal L9 L11
  constraint equal L8 L10
  measures "d222_1" distance of L8.start L8.end
  measures "d223_1" distance of L11.start L11.end
extrude "Extrude2'''''''" cut sketch "Sketch2 (6)" against normal blind 12.7 contours L4 L5 L6 L7 bodies 20 in component "right (1) (1)"
sketch "Sketch1 (14)" plane through (0, 0, 0) normal (0.707107, 0, 0.707107) x (0.707107, 0, -0.707107) in component "left (1) (1)"
  line L0 (-299.8624, 19.05) -> (-299.8624, 0)
  line L1 (-299.8624, 0) -> (-228.6, 0)
  line L2 (-228.6, 0) -> (-228.6, 19.05)
  line L3 (-228.6, 19.05) -> (-299.8624, 19.05)
  line L4 (-293.5124, 12.7) -> (-234.95, 12.7)
  line L5 (-234.95, 12.7) -> (-234.95, 6.35)
  line L6 (-234.95, 6.35) -> (-293.5124, 6.35)
  line L7 (-293.5124, 6.35) -> (-293.5124, 12.7)
  line L8 (-234.95, 8.376) -> (-228.6, 8.376) construction
  line L9 (-293.5124, 9.5249) -> (-299.8624, 9.5249) construction
  line L10 (-284.8839, 19.05) -> (-284.8839, 12.7) construction
  line L11 (-271.78, 6.35) -> (-271.78, 0) construction
  dimension "d226_1" = 6.35
  dimension "d227_1" = 6.35
  dimension "d247_1" = 58.5624
  dimension "d248_1" = 6.35
  constraint horizontal L4
  constraint vertical L5
  constraint horizontal L6
  constraint vertical L7
  constraint coincident L5 L8.start
  constraint perpendicular L5 L8
  constraint coincident L7 L9.start
  constraint coincident L0 L9.end
  constraint perpendicular L0 L9
  constraint coincident L3 L10.start
  constraint coincident L4 L10.end
  constraint perpendicular L4 L10
  constraint coincident L6 L11.start
  constraint coincident L1 L11.end
  constraint perpendicular L1 L11
  constraint equal L10 L11
  constraint equal L8 L9
  constraint coincident L2 L8.end
  measures "d226_1" distance of L9.start L9.end
  measures "d227_1" distance of L10.start L10.end
  measures "d247_1" distance of L4.start L4.end
  measures "d248_1" distance of L4.start L6.end
extrude "Extrude1'''''''''''''" cut sketch "Sketch1 (14)" against normal blind 12.7 contours L4 L5 L6 L7 bodies 23 in component "left (1) (1)"